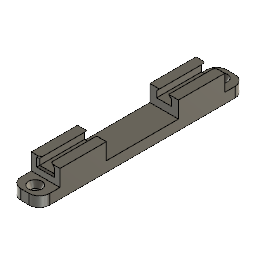
dsi-base-upright (Autodesk Fusion 360 design; units mm, degrees)
Autodesk Fusion 360 part; units mm, degrees
note: some values were not read from the file. Set by a fixed rule: which sketch regions a step uses.
sketch "Sketch1" plane through (0, 0, 0) normal (0, 1, 0) x (1, 0, 0)
  line L0 (-7, -13) -> (7, -13)
  line L1 (7, -13) -> (7, 0)
  line L2 (7, 0) -> (-7, 0)
  line L3 (-7, 0) -> (-7, -13)
  line L4 (-3.5, -13) -> (3.5, -13) construction
  line L5 (3.5, -13) -> (3.5, -8.75) construction
  line L6 (3.5, -8.75) -> (-3.5, -8.75) construction
  line L7 (-3.5, -8.75) -> (-3.5, -13) construction
  line L8 (-3.5, -11.75) -> (-2.25, -13) construction
  line L9 (2.25, -13) -> (3.5, -11.75) construction
  line L10 (0, -8.75) -> (0, 0) construction
  dimension "d3" = 7
  dimension "d4" = 1.25
  dimension "d5" = 1.25
  dimension "d6" = 3
  dimension "d7" = 45
  dimension "d8" = 3.5
  dimension "d9" = 3.5
  dimension "d10" = 13
  constraint horizontal L0
  constraint horizontal L2
  constraint midpoint L10.end L2
  constraint horizontal L4
  constraint vertical L5
  constraint horizontal L6
  constraint vertical L7
  constraint coincident L0 L4.start
  constraint coincident L7 L8.start
  constraint coincident L0 L8.end
  constraint coincident L4 L9.start
  constraint coincident L5 L9.end
  constraint equal L8 L9
  constraint midpoint L6 L10.start
  constraint coincident L10.end origin
  constraint vertical L10
  constraint vertical L3
  measures "d3" distance of L5.end L6.end
  measures "d4" distance of L4.start L8.end
  measures "d5" distance of L4.end L9.start
  measures "d6" distance of L5.end L9.end
  measures "d7" angle of L5 L9
  measures "d8" distance of L0.start L4.start
  measures "d9" distance of L0.end L4.end
  measures "d10" distance of L0 L2
extrude "Extrude1" add sketch "Sketch1" along normal mid plane 80
sketch "Sketch2" plane through (0, 0, 0) normal (0, 0, 1) x (1, 0, 0)
  line L0 (-7, -40) -> (7, -40)
  line L1 (7, -40) -> (7, -45)
  line L2 (2, -50) -> (-2, -50)
  line L3 (-7, -45) -> (-7, -40)
  arc A0 (2, -50) -> (7, -45) centre (2, -45) ccw
  arc A1 (-7, -45) -> (-2, -50) centre (-2, -45) ccw
  line L4 (7, -40) -> (-7, -40)
  point P0 (7, -50)
  dimension "d13" = 10
  dimension "d14" = 5
  constraint horizontal L0
  constraint vertical L1
  constraint horizontal L2
  constraint vertical L3
  constraint coincident P0 L1
  constraint coincident P0 L2
  constraint tangent L1 A0
  constraint tangent L2 A0
  constraint tangent L2 A1
  constraint tangent L3 A1
  constraint equal A0 A1
  constraint equal L0 L4
  constraint midpoint L0 L4
  measures "d13" distance of L0.end P0
  measures "d14" radius of A0
extrude "Extrude2" add sketch "Sketch2" along normal blind 5
sketch "Sketch3" plane through (0, 0, 5) normal (0, 0, 1) x (-1, 0, 0)
  line L0 (7, 40) -> (7, 45)
  arc A0 (7, 45) -> (2, 50) centre (2, 45) ccw
  line L1 (2, 50) -> (-2, 50)
  arc A1 (-2, 50) -> (-7, 45) centre (-2, 45) ccw
  line L2 (-7, 45) -> (-7, 40)
  line L3 (-7, 40) -> (7, 40)
  circle A2 centre (0, 45) radius 1.75
  line L4 (-7, 45) -> (7, 45) construction
  dimension "d20" = 3.5
  constraint coincident A1.end L2.start
  constraint coincident L0.end A0.start
  constraint midpoint A2.centre L4
  measures "d20" diameter of A2
extrude "Extrude3" cut sketch "Sketch3" against normal blind 5 contours A2
chamfer "Chamfer1" distance 1.5 angle 60 1 edges at (1.6316, -45.6328, 5) measured on face at (-5.1922, -43.0802, 5)
mirror "Mirror1" about plane through (0, 0, 0) normal (0, 1, 0) of "Extrude2", "Extrude3", "Chamfer1"
sketch "Sketch4" plane through (0, -40, 0) normal (0, -1, 0) x (1, 0, 0)
  line L0 (-7, 5) -> (7, 5)
  line L1 (7, 5) -> (7, 13)
  line L2 (7, 13) -> (-7, 13)
  line L3 (-7, 13) -> (-7, 5)
  line L4 (-3.5, 8.75) -> (-3.5, 13) construction
  line L5 (-3.5, 11.75) -> (-2.25, 13) construction
  line L6 (2.25, 13) -> (3.5, 11.75) construction
  line L7 (3.5, 13) -> (3.5, 8.75) construction
  line L8 (3.5, 8.75) -> (-3.5, 8.75) construction
  line L9 (3.6, 13) -> (3.6, 8.65)
  line L10 (3.6, 8.65) -> (-3.6, 8.65)
  line L11 (-3.6, 8.65) -> (-3.6, 13)
  line L12 (-2.25, 13) -> (-3.6, 11.65)
  line L13 (2.25, 13) -> (3.6, 11.65)
  dimension "d25" = -0.1
  constraint coincident L5.end L12.start
  constraint coincident L11 L12.end
  constraint parallel L5 L12
  constraint coincident L6.start L13.start
  constraint coincident L9 L13.end
  constraint parallel L6 L13
extrude "Extrude4" cut sketch "Sketch4" against normal up to surface (80 mm away) contours L2 L9 L10 L11 L12 L13
sketch "Sketch5" plane through (-7, 0, 0) normal (-1, 0, 0) x (0, -1, 0)
  line L0 (40, 13) -> (-40, 13)
  line L1 (-40, 13) -> (-40, 5)
  line L2 (-40, 5) -> (-45, 5)
  line L3 (-45, 5) -> (-45, 0)
  line L4 (-45, 0) -> (45, 0)
  line L5 (45, 0) -> (45, 5)
  line L6 (45, 5) -> (40, 5)
  line L7 (40, 5) -> (40, 13)
  line L8 (-17.5, 13) -> (17.5, 13)
  line L9 (17.5, 13) -> (17.5, 5)
  line L10 (17.5, 5) -> (-17.5, 5)
  line L11 (-17.5, 5) -> (-17.5, 13)
  line L12 (0, 0) -> (0, 5) construction
  dimension "d28" = 35
  constraint horizontal L8
  constraint vertical L9
  constraint horizontal L10
  constraint vertical L11
  constraint coincident L0 L8.start
  constraint coincident L12.start origin
  constraint midpoint L10 L12.end
  constraint vertical L12
  constraint coincident L6.end L10
  measures "d28" distance of L9.end L10.end
extrude "Extrude5" cut sketch "Sketch5" against normal up to surface (14 mm away) contours L0 L8 L9 L10 L11
chamfer "Chamfer2" distance 0.75 angle 45 10 edges at (-2.925, -40, 12.325) (-3.6, -40, 10.15) (0, -40, 8.65) (3.6, -40, 10.15) (2.925, -40, 12.325) (2.925, 40, 12.325) (3.6, 40, 10.15) (0, 40, 8.65) (-3.6, 40, 10.15) (-2.925, 40, 12.325)
